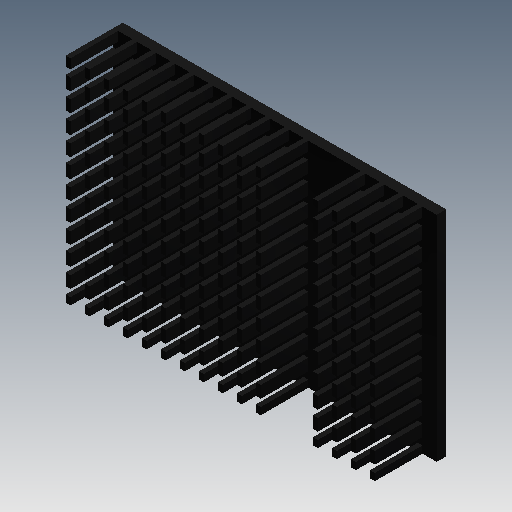
# Autodesk Inventor part: config - graphic card heat sink
Saved by Autodesk Inventor 2020 (Build 240152000, 152)
## iProperties
Created: 2005-12-11
Part Number: config - graphic card heat sink
Document SubType Name: Modeling
Designer: Simon.Ng@autodesk.com
Stock Number: config - graphic card heat sink
Density: 1 g/cm^3
Material: Generic
Mass: 10.395 g
Surface Area: 187.22 cm^2
Volume: 10.395 cm^3
Appearance: Glossy - Black
Company: Autodesk Asia Pte. Ltd.
Title: PC Demo
Author: Simon.Ng@autodesk.com
Autodesk Inventor part; units mm, degrees
ref_plane "YZ Plane" through (0, 0, 0) normal (1, 0, 0) x (0, 1, 0)
ref_plane "XZ Plane" through (0, 0, 0) normal (0, 1, 0) x (-1, 0, 0)
ref_plane "XY Plane" through (0, 0, 0) normal (0, 0, 1) x (1, 0, 0)
sketch "Sketch1" plane through (0, 0, 0) normal (0, 0, 1) x (1, 0, 0)
  line L0 (0, 36) -> (0, -27) projected
  line L1 (-40.8, 0) -> (54.4, 0) projected
  line L2 (-34, 22.5) -> (34, 22.5)
  line L3 (34, 22.5) -> (34, -22.5)
  line L4 (34, -22.5) -> (-34, -22.5)
  line L5 (-34, -22.5) -> (-34, 22.5)
  dimension "d0" = 68
  dimension "d1" = 45
  constraints: 8 end point, 2 parallel, 1 horizontal, 1 perpendicular, 2 other
  measures "d0" distance of L2.start L2.end
  measures "d1" distance of L4.end L2.start
extrude "Extrusion1" add sketch "Sketch1" along normal blind 12
sketch "Sketch3" plane through (-34, -22.5, 0) normal (0, -1, 0) x (1, 0, 0)
  line L0 (68, 12) -> (0, 12) projected
  line L1 (0, 0) -> (0, 12) projected
  line L2 (68, 0) -> (0, 0) projected
  line L3 (1, 12) -> (4, 12)
  line L4 (4, 12) -> (4, 2)
  line L5 (4, 2) -> (1, 2)
  line L6 (1, 2) -> (1, 12)
  dimension "d11" = 2
  dimension "d12" = 1
  dimension "d13" = 3
  constraints: 8 end point, 2 parallel, 1 horizontal, 1 perpendicular, 1 point on line
  measures "d11" distance between parallel lines of L2 L5
  measures "d12" distance between parallel lines of L1 L6
  measures "d13" distance of L4.end L5.end
extrude "Extrusion3" cut sketch "Sketch3" against normal through all
pattern_linear "Rectangular Pattern2" count 18 spacing 4 along (1, 0, 0) of "Extrusion3"
sketch "Sketch4" plane through (-34, -22.5, 0) normal (0, -1, 0) x (1, 0, 0)
  line L0 (49, 12) -> (41, 12)
  line L1 (41, 12) -> (41, 2)
  line L2 (41, 2) -> (49, 2)
  line L3 (49, 2) -> (49, 12)
  constraints: 8 end point, 2 parallel, 1 horizontal, 1 perpendicular
extrude "Extrusion4" cut sketch "Sketch4" against normal through all
sketch "Sketch5" plane through (0, 0, 12) normal (0, 0, 1) x (1, 0, 0)
  line L0 (31, -22.5) -> (31, 22.5) projected
  line L1 (-34, -22.5) -> (-34, 22.5) projected
  line L2 (31, 20.5) -> (-34, 20.5)
  line L3 (-34, 20.5) -> (-34, 19)
  line L4 (-34, 19) -> (31, 19)
  line L5 (31, 19) -> (31, 20.5)
  line L6 (27, 22.5) -> (30, 22.5) projected
  dimension "d21" = 2
  dimension "d22" = 1.5
  constraints: 8 end point, 2 parallel, 2 point on line, 1 horizontal, 1 perpendicular
  measures "d21" distance between parallel lines of L2 L6
  measures "d22" distance between parallel lines of L4 L2
extrude "Extrusion5" cut sketch "Sketch5" against normal up to surface (10 mm away)
pattern_linear "Rectangular Pattern3" count 12 spacing 4 along (0, -1, 0) of "Extrusion5"
body "Solid1"
